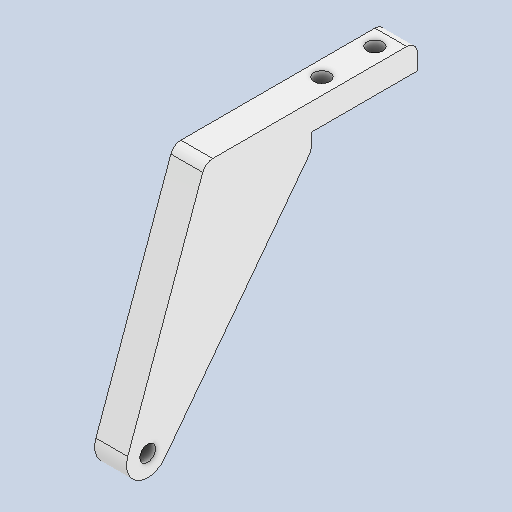
# Autodesk Inventor part: hand-grab-v1-POM-link-F-1
Saved by Autodesk Inventor 2025.1 (Build 291241000, 241)
## iProperties
Created: 2024-10-07
Part Number: hand-grab-v1-POM-link-F-1
Material: ABS プラスチック
Document SubType Name: Modeling
Designer: haruy
Density: 1.06 g/cm^3
Appearance: 白
Author: haruy
Autodesk Inventor part; units mm, degrees
ref_plane "YZ Plane" through (0, 0, 0) normal (1, 0, 0) x (0, 1, 0)
ref_plane "XZ Plane" through (0, 0, 0) normal (0, 1, 0) x (-1, 0, 0)
ref_plane "XY Plane" through (0, 0, 0) normal (0, 0, 1) x (1, 0, 0)
derived "hand-grab-v1-Sketch-Base.ipt"
sketch "スケッチ1" plane through (400, 0, 0) normal (1, 0, 0) x (0, 1, 0)
  circle A0 centre (0, 0) radius 120
  circle A1 centre (-109.5522, 63.25) radius 6.5
  line L0 (0, 0) -> (-109.5522, 63.25)
  line L1 (0, 0) -> (0, 120)
  line L2 (246.0862, 200) -> (-251.4603, 200)
  circle A2 centre (145, 60) radius 254.573
  circle A3 centre (-67.6203, 200) radius 6.5
  line L3 (0, 0) -> (-120, 0)
  line L4 (249, 9.15) -> (187, 9.15)
  line L5 (187, 9.15) -> (187, -9.15)
  line L6 (187, -9.15) -> (249, -9.15)
  line L7 (249, -9.15) -> (249, 9.15)
  line L8 (187, 5.15) -> (179, 5.15)
  line L9 (179, 5.15) -> (179, -4.85)
  line L10 (179, -4.85) -> (187, -4.85)
  line L11 (187, -4.85) -> (187, 5.15)
  line L12 (179, 3.15) -> (174, 3.15)
  line L13 (174, 3.15) -> (174, -2.85)
  line L14 (174, -2.85) -> (179, -2.85)
  line L15 (179, -2.85) -> (179, 3.15)
  line L16 (174, 2.65) -> (159, 2.65)
  line L17 (159, 2.65) -> (159, -2.35)
  line L18 (159, -2.35) -> (174, -2.35)
  line L19 (174, -2.35) -> (174, 2.65)
  line L20 (187, 34.15) -> (184, 34.15)
  line L21 (184, 34.15) -> (184, -43.5182)
  line L22 (184, -43.5182) -> (187, -43.5182)
  line L23 (187, -43.5182) -> (187, 34.15)
  circle A4 centre (150, 65) radius 4
  circle A5 centre (150, 65) radius 14 construction
  line L24 (187, 34.15) -> (192, 34.15)
  line L25 (192, 34.15) -> (192, 14.15)
  line L26 (192, 14.15) -> (187, 14.15)
  line L27 (187, 14.15) -> (187, 34.15)
  line L28 (184, 34.15) -> (147.5804, 61.8148)
  line L29 (151.3533, 68.7641) -> (192, 54.15)
  line L30 (192, 54.15) -> (192, 34.15)
  line L31 (239.3868, 130) -> (-239.3868, 130)
  circle A6 centre (-109.5522, 63.25) radius 4
  circle A7 centre (150, 65) radius 9 construction
  line L32 (-106.0881, 61.25) -> (-113.0163, 65.25)
  line L33 (170, 36) -> (155, 36)
  circle A8 centre (155, 36) radius 5
  circle A9 centre (155, 36) radius 9
  circle A10 centre (-90.698, 156.1969) radius 6.5
  circle A11 centre (170, 36) radius 5
  line L34 (150, 65) -> (170, 36)
  circle A12 centre (170, 36) radius 9
  circle A13 centre (150, 65) radius 44.2278
  line L35 (150, 65) -> (155, 36)
  line L36 (150, 65) -> (-109.5522, 63.25)
  line L37 (-90.698, 156.1969) -> (150, 65)
  circle A14 centre (150, 65) radius 1.5
  line L38 (150, 65) -> (157.5146, 21.4152)
  circle A15 centre (150, 65) radius 35.2278
  circle A16 centre (155.9855, 30.2844) radius 9
  line L39 (168.0777, 21.2844) -> (136, 21.2844)
  line L40 (175, 3.15) -> (175, -2.85)
  point P0 (187, 14.15)
  point P1 (-60, 0)
  dimension "d15" = 3
  measures "d15" diameter of A14
sketch "スケッチ2" plane through (0, 400, 0) normal (0, 1, 0) x (-1, 0, 0)
  circle A0 centre (0, 0) radius 120
  line L0 (0, 0) -> (-331.4625, 0)
  line L1 (67.5, -116.9134) -> (-135, 0)
  circle A1 centre (0, 0) radius 5
  line L2 (0, 0) -> (67.5, 116.9134)
  line L3 (0, 0) -> (67.5, -116.9134)
  line L4 (0, 0) -> (-135, 0)
  line L5 (17.0359, 37.507) -> (12.0359, 28.8468)
  line L6 (12.0359, 28.8468) -> (15.5, 26.8468)
  line L7 (15.5, 26.8468) -> (20.5, 35.507)
  line L8 (20.5, 35.507) -> (17.0359, 37.507)
  line L9 (20.5, 35.507) -> (15.5, 26.8468)
  line L10 (15.5, 26.8468) -> (18.9641, 24.8468)
  line L11 (18.9641, 24.8468) -> (23.9641, 33.507)
  line L12 (23.9641, 33.507) -> (20.5, 35.507)
  line L13 (14.5359, 33.1769) -> (21.4641, 29.1769)
  circle A2 centre (0, 0) radius 2.65
  line L14 (16.8194, 37.632) -> (10.3194, 26.3737)
  line L15 (10.3194, 26.3737) -> (5.9893, 28.8737)
  line L16 (5.9893, 28.8737) -> (12.4893, 40.132)
  line L17 (12.4893, 40.132) -> (16.8194, 37.632)
  line L18 (28.5107, 30.882) -> (24.1806, 33.382)
  line L19 (22.0107, 19.6237) -> (28.5107, 30.882)
  line L20 (24.1806, 33.382) -> (17.6806, 22.1237)
  line L21 (17.6806, 22.1237) -> (22.0107, 19.6237)
  circle A3 centre (0, 0) radius 28.3207
  line L22 (-41, 9.25) -> (-41, 4.25)
  line L23 (-41, 4.25) -> (-28, 4.25)
  line L24 (-28, 9.25) -> (-41, 9.25)
  line L25 (-28, 4.25) -> (-28, 9.25)
  line L26 (-41, -4.25) -> (-28, -4.25)
  line L27 (-41, -9.25) -> (-41, -4.25)
  line L28 (-28, -9.25) -> (-41, -9.25)
  line L29 (-28, -4.25) -> (-28, -9.25)
  line L30 (12.4893, -40.132) -> (16.8194, -37.632)
  line L31 (16.8194, -37.632) -> (10.3194, -26.3737)
  line L32 (5.9893, -28.8737) -> (12.4893, -40.132)
  line L33 (10.3194, -26.3737) -> (5.9893, -28.8737)
  line L34 (24.1806, -33.382) -> (17.6806, -22.1237)
  line L35 (28.5107, -30.882) -> (24.1806, -33.382)
  line L36 (22.0107, -19.6237) -> (28.5107, -30.882)
  line L37 (17.6806, -22.1237) -> (22.0107, -19.6237)
  line L38 (5.9893, 28.8737) -> (5.373, 27.8064)
  line L39 (22.0107, 19.6237) -> (21.3945, 18.5564)
  line L40 (-28, 9.25) -> (-26.7675, 9.25)
  line L41 (-28, -9.25) -> (-26.7675, -9.25)
  line L42 (5.9893, -28.8737) -> (2.1934, -22.2991)
  line L43 (22.0107, -19.6237) -> (21.3945, -18.5564)
  line L44 (13.6109, 31.5748) -> (3.6109, 14.2543)
  line L45 (3.6109, 14.2543) -> (-1.5853, 17.2543)
  line L46 (-1.5853, 17.2543) -> (8.4147, 34.5748)
  line L47 (8.4147, 34.5748) -> (13.6109, 31.5748)
  circle A4 centre (3.5128, 20.0844) radius 1.5
  circle A5 centre (8.5128, 28.7446) radius 1.5
  circle A6 centre (20.6372, 21.7446) radius 1.5
  circle A7 centre (15.6372, 13.0844) radius 1.5
  circle A8 centre (-29.15, 7) radius 1.5
  circle A9 centre (-19.15, 7) radius 1.5
  circle A10 centre (-19.15, -7) radius 1.5
  circle A11 centre (-29.15, -7) radius 1.5
  circle A12 centre (8.5128, -28.7446) radius 1.5
  circle A13 centre (3.5128, -20.0844) radius 1.5
  circle A14 centre (15.6372, -13.0844) radius 1.5
  circle A15 centre (20.6372, -21.7446) radius 1.5
  line L48 (1.0128, 15.7543) -> (13.6109, 31.5748)
  circle A16 centre (0, 0) radius 34.3835
  line L49 (-8, 47) -> (-188, 47)
  line L50 (-188, 47) -> (-188, 32)
  line L51 (-188, 32) -> (-8, 32)
  line L52 (-8, 32) -> (-8, 47)
ref_plane "作業平面1" through (400, 0, 0) normal (1, 0, 0) x (0, 1, 0)
ref_plane "作業平面2" through (0, 400, 0) normal (0, 1, 0) x (-1, 0, 0)
extrude "押し出し1" add sketch "スケッチ1" along normal blind 6 contours L36 A14 L35 A4 | A4 L37 A14 L36 | A13 L28 A12 A15 L29 L30 | L30 L24 L20 L28 A13 | A4 L34 A14 L37 | A4 L35 L28 | A14 L37 L36 | L36 L35 A14 | L25 L26 L23 L24 | L29 A15 A12 L28 L34 A4 | A14 L34 L37 | L35 A14 L34 A4 | A4 L34 L28 L35 | L34 A14 L35 | L28 A15 A12 | A15 L28 A12
sketch "スケッチ3" plane through (400, 192, 54.15) normal (0, 1, 0) x (1, 0, 0)
  line L0 (0, 40) -> (6, 40) projected
  line L1 (6, 40) -> (6, 0) projected
  point P0 (-400, 54.15)
  point P1 (3, 25)
  point P2 (3, 35)
  dimension "d3" = 5
  dimension "d4" = 10
  dimension "d5" = 3
  dimension "d6" = 3
  measures "d3" distance from line of point (3, 35) L0
  measures "d4" distance of point (3, 25) point (3, 35)
  measures "d5" distance from line of point (3, 25) L1
  measures "d6" distance from line of point (3, 35) L1
hole "穴1" at (403, 192, 29.15) at (403, 192, 19.15) direction (0, -1, 0) diameter 3 end through all
fillet "フィレット1" radius 2 3 edges at (403, 192, 54.15) (403, 192, 14.15) (403, 184, 34.15)
extrude "押し出し2" cut sketch "スケッチ1" along normal blind 6 contours A14 L37 L36 | L36 L35 A14 | A14 L34 L37 | L34 A14 L35
sketch "スケッチ4" plane through (406, 187, 34.15) normal (1, 0, 0) x (0, 0, -1)
  line L0 (-35.6293, -41.3898) -> (25.2709, -41.3898)
  line L1 (25.2709, -41.3898) -> (25.2709, 5.8521)
  line L2 (25.2709, 5.8521) -> (-35.6293, 5.8521)
  line L3 (-35.6293, 5.8521) -> (-35.6293, -41.3898)
  point P0 (34.15, -187)
  dimension "d18" = 60.9003
  dimension "d19" = 47.2419
  constraints: 8 end point, 2 parallel, 1 horizontal, 1 perpendicular
  measures "d18" distance of L1.end L2.end
  measures "d19" distance of L0.end L1.end
sketch "スケッチ5" plane through (406, 187, 34.15) normal (1, 0, 0) x (0, 0, -1)
  circle A0 centre (-30.85, -37) radius 1.5 projected
  arc A1 (-0.4074, -3.5363) -> (0, -2.3265) centre (-2, -2.3265) ccw projected
  line L0 (0, -2.3265) -> (0, 0) projected
  line L1 (0, 0) -> (20, 0) projected
  line L2 (20, 0) -> (20, 3) projected
  arc A2 (20, 3) -> (18, 5) centre (18, 3) ccw projected
  line L3 (18, 5) -> (-18.5937, 5) projected
  arc A3 (-18.5937, 5) -> (-20.4758, 3.6767) centre (-18.5937, 3) ccw projected
  line L4 (-20.4758, 3.6767) -> (-34.6141, -35.6467) projected
  arc A4 (-34.6141, -35.6467) -> (-27.6648, -39.4196) centre (-30.85, -37) ccw projected
  line L5 (-27.6648, -39.4196) -> (-0.4074, -3.5363) projected
  point P0 (34.15, -187)
equation "\"d6\" = d5"
